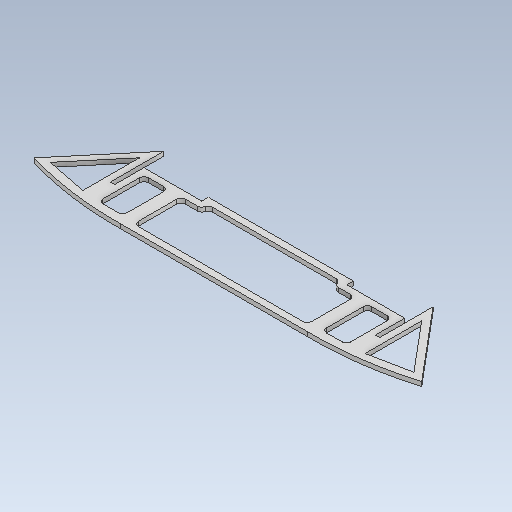
# Autodesk Inventor part: bulkhead_B1
Saved by Autodesk Inventor 2020.3 (Build 243373010, 373A)
## iProperties
Created: 2020-05-22
Part Number: bulkhead_B1
Material: Generic
Document SubType Name: Modeling
Designer: kardo
Density: 1 g/cm^3
Appearance: Default
Mass: 3.64799 g
Surface Area: 55.8545 cm^2
Volume: 3.64799 cm^3
Author: kardo
Autodesk Inventor part; units mm, degrees
ref_plane "YZ Plane" through (0, 0, 0) normal (1, 0, 0) x (0, 1, 0)
ref_plane "XZ Plane" through (0, 0, 0) normal (0, 1, 0) x (-1, 0, 0)
ref_plane "XY Plane" through (0, 0, 0) normal (0, 0, 1) x (1, 0, 0)
derived "base_sketch.ipt"
sketch "bulkhead_B1" plane through (0, -102, 0) normal (0, 1, 0) x (-1, 0, 0)
  line L0 (19.176, 46.818) -> (62.322, 46.818)
  line L1 (0, 19.935) -> (0, 0)
  line L2 (62.322, 46.818) -> (62.322, 13.529)
  line L3 (0, 5.6919) -> (-27.3644, 38.3035)
  line L4 (62.322, 44.7066) -> (19.176, 44.7066)
  line L5 (-38.352, 36.72) -> (-38.352, 34.6086) construction
  line L6 (-19.176, 42.5952) -> (-19.176, 40.4838) construction
  line L7 (0, 45.9) -> (0, 43.7886) construction
  line L8 (19.176, 46.818) -> (19.176, 44.7066) construction
  line L9 (0, 19.935) -> (28.764, 19.935)
  line L10 (28.764, 19.935) -> (28.764, 13.529)
  line L11 (28.764, 13.529) -> (62.322, 13.529)
  line L12 (62.322, 13.7901) -> (28.764, 13.7901)
  line L13 (28.764, 13.7901) -> (28.764, 16.8245)
  line L14 (28.764, 16.8245) -> (0, 16.8245)
  line L15 (0, 16.8245) -> (0, 5.6919)
  spline S0 degree 4 poles (-57.528, 27.54) (-46.0483, 34.2051) (-30.6129, 40.5281) (-11.2214, 45.0414) (8.3201, 46.818) (15.5662, 46.818) (19.176, 46.818) knots 0 0 0 0 0 0.630279 0.815816 1 1 1 1 1
  spline S1 degree 3 poles (19.176, 44.7066) (-0.1981, 44.9447) (-19.6083, 41.6917) (-38.352, 34.6086) knots 0 0 0 0 1 1 1 1
  point P0 (0, 3.825)
  point P1 (0, 13.7901)
ref_plane "bulkhead_B1_plane" through (0, -102, 0) normal (0, 1, 0) x (-1, 0, 0)
sketch "Sketch2" plane through (0, -102, 0) normal (0, 1, 0) x (-1, 0, 0)
  spline S0 degree 3 poles (19.176, 44.7066) (-0.1981, 44.9447) (-19.6083, 41.6917) (-38.352, 34.6086) knots 0 0 0 0 1 1 1 1 projected
  line L0 (62.322, 44.7066) -> (19.176, 44.7066) projected
  line L1 (62.322, 46.818) -> (62.322, 13.529) projected
  line L2 (0, 5.6919) -> (-27.3644, 38.3035) projected
  line L3 (0, 16.8245) -> (0, 3.825) projected
  line L4 (28.764, 16.8245) -> (0, 16.8245) projected
  line L5 (28.764, 13.7901) -> (28.764, 16.8245) projected
  line L6 (62.322, 13.7901) -> (28.764, 13.7901) projected
  line L7 (-21.8143, 36.3564) -> (-3, 13.9343)
  line L8 (-3, 13.9343) -> (-3, 40.1276)
  line L9 (-3, 40.1276) -> (-21.8143, 36.3564)
  line L10 (5, 38.7886) -> (5, 21.8245)
  line L11 (7, 19.8245) -> (14.176, 19.8245)
  line L12 (16.176, 21.8245) -> (16.176, 38.7886)
  line L13 (14.176, 40.7886) -> (7, 40.7886)
  line L14 (22.176, 39.7066) -> (22.176, 21.8245)
  line L15 (24.176, 19.8245) -> (29.8231, 19.8245)
  line L16 (33.7049, 16.7901) -> (62.322, 16.7901)
  line L17 (62.322, 41.7066) -> (24.176, 41.7066)
  line L18 (0, 16.8245) -> (0, 30.3066)
  line L19 (-27.3644, 38.3035) -> (0, 43.7886) construction
  arc A0 (16.176, 38.7886) -> (14.176, 40.7886) centre (14.176, 38.7886) ccw
  arc A1 (7, 40.7886) -> (5, 38.7886) centre (7, 38.7886) ccw
  arc A2 (5, 21.8245) -> (7, 19.8245) centre (7, 21.8245) ccw
  arc A3 (14.176, 19.8245) -> (16.176, 21.8245) centre (14.176, 21.8245) ccw
  arc A4 (22.176, 21.8245) -> (24.176, 19.8245) centre (24.176, 21.8245) ccw
  arc A5 (24.176, 41.7066) -> (22.176, 39.7066) centre (24.176, 39.7066) ccw
  arc A6 (31.764, 18.3073) -> (29.8231, 19.8245) centre (29.8231, 17.8245) ccw
  arc A7 (31.764, 18.3073) -> (33.7049, 16.7901) centre (33.7049, 18.7901) ccw
  line L20 (0, 30.3066) -> (0, 43.7886) construction
  line L21 (0, 30.3066) -> (2, 30.3066)
  line L22 (2, 30.3066) -> (2, 16.6552)
  point P0 (0, 0)
  point P1 (5, 40.7886)
  point P2 (22.176, 41.7066)
  point P3 (2, 16.8245)
  dimension "d1" = 3
  dimension "d2" = 3
  dimension "d4" = 3
  dimension "d6" = 3
  dimension "d7" = 3
  dimension "d8" = 3
  dimension "d9" = 3
  dimension "d10" = 3
  dimension "d11" = 3
  dimension "d13" = 3
  dimension "d14" = 2
  dimension "d16" = 2
  dimension "d17" = 3
  dimension "d20" = 3
  dimension "d21" = 2
  constraints: 32 end point, 16 point on circle, 15 tangent, 11 parallel, 8 centre point, 6 equal radius, 6 point on line, 3 collinear, 1 perpendicular, 3 other
  measures "d2" distance between parallel lines of L3 L8
  measures "d4" distance between parallel lines of L4 L11
  measures "d6" vertical distance of point (5, 40.789) L19.end
  measures "d7" distance from line of L0.end L12
  measures "d8" horizontal distance of point (22.176, 41.707) L0.end
  measures "d9" distance between parallel lines of L0 L17
  measures "d10" distance between parallel lines of L4 L15
  measures "d11" distance between parallel lines of L6 L16
  measures "d13" distance between parallel lines of L19 L9
  measures "d14" radius of A0
  measures "d16" radius of A6
  measures "d17" distance from line of L5 A6.start
  measures "d20" distance between parallel lines of L10 L22
  measures "d21" distance between parallel lines of L22 L18
extrude "Extrusion1" add sketch "Sketch2" along normal blind 2 contours L0 L1 L17 A5 L14 A4 L15 A6 A7 L16 L6 L5 L4 L22 L21 L18 L3 L2 S0
mirror "Mirror1" about plane through (-62.322, -102, 13.7901) normal (-1, 0, 0) of "Extrusion1"
equation "\"d21\" = stringer_thickness"
equation "\"d18\" = bulkhead_thickness"
equation "\"stringer_thickness\" = 2"
equation "\"bulkhead_thickness\" = 2"
body "Solid1"
